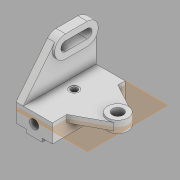
# Autodesk Inventor part: Bracket Support
Saved by Autodesk Inventor 2020 (Build 240168000, 168)
## iProperties
Created: 2019-09-11
Part Number: Bracket Support
Material: Generic
Document SubType Name: Modeling
Designer: Jorge
Density: 1 g/cm^3
Appearance: Default
Author: Jorge
Autodesk Inventor part; units mm, degrees
ref_plane "YZ Plane" through (0, 0, 0) normal (1, 0, 0) x (0, 1, 0)
ref_plane "XZ Plane" through (0, 0, 0) normal (0, 1, 0) x (-1, 0, 0)
ref_plane "XY Plane" through (0, 0, 0) normal (0, 0, 1) x (1, 0, 0)
sketch "Sketch1" plane through (0, 0, 0) normal (0, 0, 1) x (1, 0, 0)
  line L0 (-11, -17.4) -> (11, -17.4)
  line L1 (25, -12.6) -> (25, 12.6)
  line L2 (25, 12.6) -> (-25, 12.6)
  line L3 (-25, 12.6) -> (-25, -12.6)
  line L4 (-25.624, -12.9145) -> (25, 12.6) construction
  line L5 (30.644, -15.4446) -> (-25, 12.6) construction
  line L6 (11, -17.4) -> (11, -12.6)
  line L7 (0, -23.4) -> (0, 18.6) construction
  line L8 (-11, -12.6) -> (-11, -17.4)
  line L9 (-25, -12.6) -> (-11, -12.6)
  line L10 (11, -12.6) -> (25, -12.6)
  line L11 (-36.8776, 0) -> (41.8976, 0) construction
  point P0 (0, 0)
  point P1 (0, -17.4)
  point P2 (25, 0)
  point P3 (0, 0)
  dimension "d0" = 50
  dimension "d2" = 22
  dimension "d4" = 4.8
  dimension "d5" = 30
  constraints: 20 end point, 4 point on line, 3 horizontal, 2 equal length, 2 midpoint, 2 parallel, 2 vertical, 1 coincident, 1 perpendicular
  measures "d0" distance of L2.end L1.end
  measures "d2" distance between parallel lines of L6 L8
  measures "d4" distance between parallel lines of L10 L0
  measures "d5" distance between parallel lines of L2 L0
extrude "Extrusion1" add sketch "Sketch1" along normal mid plane 100
sketch "Sketch2" plane through (-25, -12.6, 50) normal (-1, 0, 0) x (0, 0, 1)
  line L0 (-100, 25.2) -> (0, 25.2) projected
  line L1 (0, 25.2) -> (-43.265, 79.5428)
  line L2 (-55, 85.2) -> (-85, 85.2)
  line L3 (-100, 70.2) -> (-100, 25.2)
  arc A0 (-43.265, 79.5428) -> (-55, 85.2) centre (-55, 70.2) ccw
  arc A1 (-85, 85.2) -> (-100, 70.2) centre (-85, 70.2) ccw
  line L4 (0, 25.2) -> (0, 0) construction
  line L5 (-85, 70.2) -> (-55, 70.2) construction
  point P0 (-50, 12.6)
  dimension "d9" = 55
  dimension "d10" = 15
  dimension "d11" = 45
  constraints: 8 end point, 4 point on circle, 4 tangent, 2 centre point, 2 horizontal, 1 equal radius, 1 perpendicular
  measures "d9" distance from line of L4 A0.centre
  measures "d10" radius of A1
  measures "d11" distance between parallel lines of L5 L0
extrude "Extrusion2" add sketch "Sketch2" against normal blind 10
sketch "Sketch3" plane through (25, 12.6, 50) normal (0, 1, 0) x (1, 0, 0)
  line L0 (0, 100) -> (0, 0) construction
  line L1 (0, 100) -> (0, 0) construction
  line L2 (0, 20) -> (41.6953, 42.7047)
  arc A0 (41.6953, 42.7047) -> (49, 55) centre (35, 55) ccw
  line L3 (0, 0) -> (-40, 0) construction
  line L4 (-50, 100) -> (-50, 85) construction
  line L5 (13.506, 55) -> (79.1808, 55) construction
  line L6 (0, 90) -> (41.6953, 67.2953)
  arc A1 (49, 55) -> (41.6953, 67.2953) centre (35, 55) ccw
  line L7 (0, 90) -> (0, 20)
  point P0 (-25, 50)
  dimension "d15" = 55
  dimension "d16" = 14
  dimension "d17" = 35
  dimension "d18" = 85
  constraints: 8 end point, 4 point on circle, 2 centre point, 2 point on line, 2 symmetric about line, 1 collinear, 1 horizontal, 1 tangent, 1 other
  measures "d15" distance from line of A0.centre L3
  measures "d16" radius of A0
  measures "d17" horizontal distance of A0.centre L2.start
  measures "d18" distance from line of A0.centre L4
extrude "Extrusion3" add sketch "Sketch3" against normal blind 10
ref_plane "Work Plane1" through (-15, 7.6, 50) normal (0, 1, 0) x (1, 0, 0)
sketch "Sketch4" plane through (-15, 7.6, 50) normal (0, 1, 0) x (1, 0, 0)
  arc A0 (81.6953, 42.7047) -> (81.6953, 67.2953) centre (75, 55) ccw projected
  circle A1 centre (75, 55) radius 14
  point P0 (15, 50)
  point P1 (81.6953, 42.7047)
  constraints: 1 centre point, 1 coincident
extrude "Extrusion4" add sketch "Sketch4" along normal mid plane 16
sketch "Sketch5" plane through (-15, -12.6, 50) normal (1, 0, 0) x (0, 0, -1)
  line L0 (55, 70.2) -> (85, 70.2) construction
  line L1 (55, 55.2) -> (85, 55.2)
  line L2 (85, 85.2) -> (55, 85.2)
  arc A0 (55, 85.2) -> (55, 55.2) centre (55, 70.2) ccw
  arc A1 (85, 55.2) -> (85, 85.2) centre (85, 70.2) ccw
  arc A2 (100, 70.2) -> (85, 85.2) centre (85, 70.2) ccw construction
  line L3 (85, 85.2) -> (55, 85.2) construction
  point P0 (50, 12.6)
  point P1 (70, 70.2)
  dimension "d24" = 30
  constraints: 8 end point, 4 point on circle, 4 tangent, 2 centre point, 2 concentric, 1 horizontal, 1 midpoint, 1 parallel
  measures "d24" distance of L0.start L0.end
extrude "Extrusion5" add sketch "Sketch5" along normal blind 3
sketch "Sketch6" plane through (-12, -12.6, 50) normal (1, 0, 0) x (0, 0, -1)
  point P0 (50, 12.6)
sketch "Boceto7" plane through (-12, -12.6, 50) normal (1, 0, 0) x (0, 0, -1)
  line L0 (55, 70.5168) -> (85, 70.5168) construction
  line L1 (55, 64.1668) -> (85, 64.1668)
  line L2 (85, 76.8668) -> (55, 76.8668)
  arc A0 (55, 76.8668) -> (55, 64.1668) centre (55, 70.5168) ccw
  arc A1 (85, 64.1668) -> (85, 76.8668) centre (85, 70.5168) ccw
  line L3 (100, 25.2) -> (100, 70.2) projected
  line L4 (0, 0) -> (0, 25.2) projected
  point P0 (50, 12.6)
  point P1 (70, 70.5168)
  dimension "d27" = 15
  dimension "d30" = 30
  dimension "d33" = 55
  dimension "d35" = 12.7
  constraints: 8 end point, 4 point on circle, 4 tangent, 2 centre point, 1 horizontal, 1 midpoint, 1 parallel
  measures "d27" distance of point (70, 70.517) L0.end
  measures "d30" distance of L0.end L0.start
  measures "d33" distance from line of L4 L0.start
  measures "d35" distance between parallel lines of L1 L2
extrude "AgujeroSuperior" cut sketch "Boceto7" against normal blind 13
sketch "Boceto8" plane through (0, 0, 50) normal (0, 0, 1) x (1, 0, 0)
  line L0 (-11, -17.4) -> (11, -17.4) projected
  circle A0 centre (0, -1.4) radius 6.25
  line L1 (-11, -12.6) -> (-11, -17.4) projected
  point P0 (0, 0)
  dimension "d37" = 12.5
  dimension "d38" = 11
  dimension "d39" = 16
  constraints: 1 centre point
  measures "d37" diameter of A0
  measures "d38" distance from line of L1 A0.centre
  measures "d39" distance from line of L0 A0.centre
extrude "AgujeroFrontal" cut sketch "Boceto8" against normal blind 100
sketch "Boceto10" plane through (60, 15.6, -5) normal (0, 1, 0) x (1, 0, 0)
  circle A0 centre (0, 0) radius 7.5
  circle A1 centre (0, 0) radius 14 construction
  point P0 (-60, -5)
  dimension "d47" = 15
  dimension "d48" = 28
  constraints: 1 centre point
  measures "d47" diameter of A0
  measures "d48" diameter of A1
extrude "AgujeroCirculo" cut sketch "Boceto10" against normal blind 16
sketch "Boceto11" plane through (-15, 12.6, -50) normal (0, 1, 0) x (1, 0, 0)
  circle A0 centre (15, -45) radius 6.5 construction
  line L0 (40, -10) -> (40, -80) construction
  point P0 (15, -50)
  dimension "d52" = 13
  dimension "d53" = 25
  dimension "d54" = 35
  constraints: 2 coincident, 1 centre point
  measures "d52" diameter of A0
  measures "d53" distance from line of A0.centre L0
  measures "d54" vertical distance of L0.end A0.centre
hole "Agujero1" at (0, 12.6, -5) direction (0, -1, 0) diameter 9 end through all counterbore diameter 13 counterbore depth 0.3
body "Solid1"
